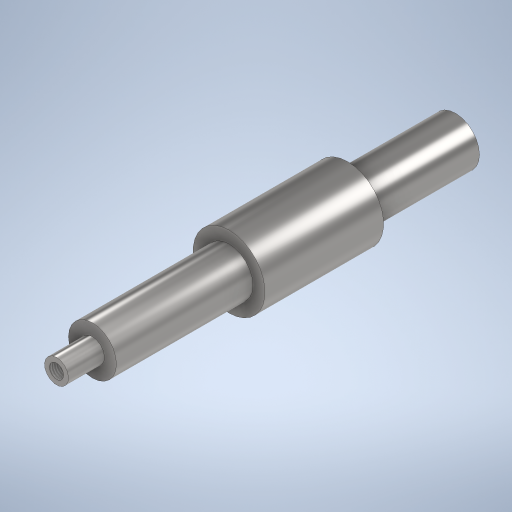
# Autodesk Inventor part: SP002
Saved by Autodesk Inventor 2023 (Build 270158000, 158)
## iProperties
Created: 2022-09-16
Part Number: SP002
Material: Steel, Mild
Document SubType Name: Modeling
Designer: D.C. Eksteen
Density: 7.85 g/cm^3
Appearance: Semi-Polished
Author: D.C. Eksteen
Title: TEST SHAFT
Autodesk Inventor part; units mm, degrees
ref_plane "YZ Plane" through (0, 0, 0) normal (1, 0, 0) x (0, 1, 0)
ref_plane "XZ Plane" through (0, 0, 0) normal (0, 1, 0) x (-1, 0, 0)
sketch "Sketch1" plane through (0, 0, 0) normal (1, 0, 0) x (0, 1, 0)
  line L0 (0, 0) -> (5, 0)
  line L1 (5, 0) -> (5, -15)
  line L2 (5, -15) -> (10, -15)
  line L3 (10, -15) -> (10, -72)
  line L4 (10, -72) -> (15, -72)
  line L5 (15, -72) -> (15, -121.5)
  line L6 (15, -121.5) -> (10, -121.5)
  line L7 (10, -121.5) -> (10, -166.5)
  line L8 (10, -166.5) -> (0, -166.5)
  line L9 (0, -166.5) -> (0, -166.5)
  line L10 (0, -166.5) -> (0, -166.5)
  line L11 (0, -166.5) -> (0, 0)
  point P0 (0, -83.25)
  point P1 (15, -96.75)
  point P2 (5, -166.5)
  point P3 (2.5, 0)
  point P4 (12.5, -72)
  dimension "d0" = 15
  dimension "d1" = 5
  dimension "d3" = 10
  dimension "d4" = 49.5
  dimension "d5" = 15
  dimension "d6" = 45
  dimension "d7" = 0
  dimension "d8" = 0
  dimension "d9" = 72
  constraints: 24 end point, 10 perpendicular, 5 midpoint, 2 point on line, 1 horizontal
  measures "d0" distance of L0.end L1.end
  measures "d1" distance between parallel lines of L11 L1
  measures "d3" distance from line of point (0, -83.25) L3
  measures "d4" distance of L4.end L5.end
  measures "d5" distance from line of L11 point (15, -96.75)
  measures "d6" distance of L6.end L7.end
  measures "d7" distance from line of point (5, -166.5) L10
  measures "d8" distance of L10.end L8.end
  measures "d9" vertical distance of point (2.5, 0) point (12.5, -72)
revolve "Revolution1" add sketch "Sketch1" angle 360 about axis through (0, 0, -166.5) along (0, 0, 1)
sketch "Sketch2" plane through (0, 0, 0) normal (0, 0, 1) x (1, 0, 0)
  circle A0 centre (0, 0) radius 5 projected
  constraints: 1 coincident
hole "Hole1" at (0, 0, 0) direction (0, 0, -1) diameter 5.9175 depth 19.1 tip angle 118 thread size "M7x1" class "6H" standard "ANSI Metric M Profile"
sketch "Sketch3" plane through (0, 0, -166.5) normal (0, 0, -1) x (-1, 0, 0)
  circle A0 centre (0, 0) radius 10 projected
  line L0 (0, 0) -> (10, 0)
  circle A1 centre (0, 0) radius 10 projected
  constraints: 2 end point, 1 horizontal, 1 horizontal alignment, 1 other
ref_plane "Work Plane1" through (-10, 0, -166.5) normal (-1, 0, 0) x (0, -1, 0)
sketch "Sketch4" plane through (-10, 0, -166.5) normal (-1, 0, 0) x (0, -1, 0)
  line L0 (10, 45) -> (-10, 45) projected
  line L1 (10, 0) -> (-10, 0) projected
  line L2 (10, 0) -> (-10, 0) projected
  line L3 (0, 0) -> (-5.5, 0)
  line L4 (-5.5, 0) -> (-5.5, 13)
  line L5 (-5.5, 13) -> (5.5, 13) construction
  line L6 (5.5, 13) -> (5.5, 0)
  line L7 (0, 0) -> (5.5, 0)
  arc A0 (5.5, 13) -> (-5.5, 13) centre (0, 13) ccw
  point P0 (0, 166.5)
  point P1 (-5.5, 0)
  dimension "d18" = 5.5
  dimension "d19" = 13
  dimension "d20" = 11
  constraints: 10 end point, 4 perpendicular, 2 midpoint, 2 point on circle, 2 point on line, 1 centre point
  measures "d18" distance of L3.start L3.end
  measures "d19" distance of L3.end L4.end
  measures "d20" distance of L4.end L5.end
extrude "Extrusion1" cut sketch "Sketch4" against normal blind 3
sketch "Sketch5" plane through (-7, -5.5, -166.5) normal (0, 0, -1) x (-1, 0, 0)
  point P0 (-7, 5.5)
  point P1 (-7, 5.5)
  constraints: 1 coincident
hole "Hole2" at (0, 0, -166.5) direction (0, 0, 1) diameter 5.9175 depth 19.1 tip angle 118 thread size "M7x1" class "6H" standard "ANSI Metric M Profile"
body "Solid1"
